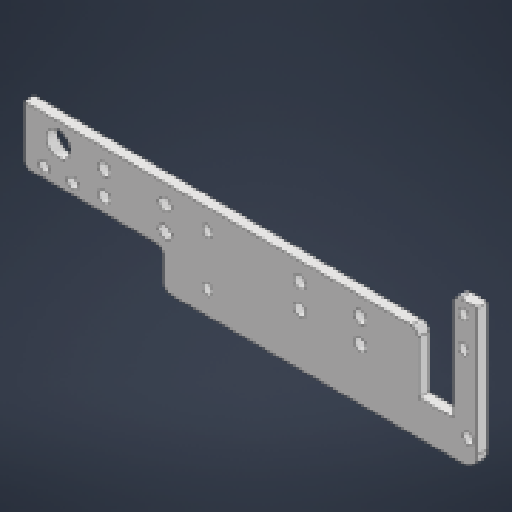
# Autodesk Inventor part: 外宽挤压
Saved by Autodesk Inventor 2025 (Build 290162000, 162)
## iProperties
Created: 2026-04-26
Part Number: 外宽挤压
Material: 常规
Document SubType Name: Modeling
Designer: XH
Density: 1 g/cm^3
Appearance: 默认
Author: XH
Autodesk Inventor part; units mm, degrees
ref_plane "YZ Plane" through (0, 0, 0) normal (1, 0, 0) x (0, 1, 0)
ref_plane "XZ Plane" through (0, 0, 0) normal (0, 1, 0) x (-1, 0, 0)
ref_plane "XY Plane" through (0, 0, 0) normal (0, 0, 1) x (1, 0, 0)
sketch "草图1" plane through (0, 0, 0) normal (0, 0, 1) x (1, 0, 0)
  line L0 (-43.79, -13.889) -> (86.21, -13.889)
  line L1 (86.21, -13.889) -> (86.21, 16.111)
  line L2 (86.21, 16.111) -> (-43.79, 16.111)
  line L3 (-43.79, 16.111) -> (-43.79, -13.889)
  dimension "d3" = 130
  dimension "d4" = 30
  constraints: 8 end point, 2 parallel, 1 horizontal, 1 perpendicular
  measures "d3" distance of L0.start L0.end
  measures "d4" distance of L0.end L1.end
extrude "拉伸1" add sketch "草图1" along normal blind 3
sketch "草图2" plane through (0, 0, 3) normal (0, 0, 1) x (1, 0, 0)
  line L0 (86.21, 16.111) -> (-43.79, 16.111) projected
  line L1 (69.2643, 16.111) -> (79.2643, 16.111)
  line L2 (79.2643, 16.111) -> (79.2643, -3.889)
  line L3 (79.2643, -3.889) -> (69.2643, -3.889)
  line L4 (69.2643, -3.889) -> (69.2643, 16.111)
  point P0 (0, 0)
  dimension "d5" = 10
  dimension "d6" = 20
  constraints: 8 end point, 2 parallel, 1 horizontal, 1 perpendicular, 1 point on line
  measures "d5" distance of L2.end L3.end
  measures "d6" distance of L1.end L2.end
extrude "拉伸2" cut sketch "草图2" against normal blind 3
fillet "圆角1" radius 2 2 edges at (69.2643, 16.111, 1.5) (79.2643, 16.111, 1.5)
sketch "草图3" plane through (0, 0, 3) normal (0, 0, 1) x (1, 0, 0)
  line L0 (-43.79, 16.111) -> (-43.79, -13.889) projected
  line L1 (-43.79, -13.889) -> (-3.79, -13.889)
  line L2 (-3.79, -13.889) -> (-3.79, 4.111)
  line L3 (-3.79, 4.111) -> (-43.79, 4.111)
  line L4 (-43.79, 4.111) -> (-43.79, -13.889)
  point P0 (0, 0)
  dimension "d10" = 40
  dimension "d11" = 18
  constraints: 8 end point, 2 parallel, 1 horizontal, 1 perpendicular
  measures "d10" distance between parallel lines of L2 L0
  measures "d11" distance between parallel lines of L1 L3
extrude "拉伸3" cut sketch "草图3" against normal blind 3
fillet "圆角2" radius 2 2 edges at (-3.79, 4.111, 1.5) (-3.79, -13.889, 1.5)
fillet "圆角3" radius 2 1 edges at (-43.79, 4.111, 1.5)
move faces "移动1" translate (0, 10.75, 0) faces at (84.5614, 16.111, 1)
fillet "圆角4" radius 4.25 1 edges at (86.21, -13.889, 1.5)
move faces "移动2" translate (0, -7.25, 0) faces at (-17.79, 4.111, 1)
sketch "草图4" plane through (0, 0, 0) normal (0, 0, -1) x (-1, 0, 0)
  line L0 (-0.892, -15.4705) -> (-0.8856, 17.0295) projected
  line L1 (-16.692, -15.4674) -> (-16.6856, 17.0326) projected
  line L2 (-0.889, 0) -> (-16.689, 0.0031)
  line L3 (-8.789, -13.6529) -> (-8.789, 16.111)
  line L4 (-67.2643, 16.111) -> (43.79, 16.111) projected
  circle A0 centre (-8.789, -7.1669) radius 1.55
  circle A1 centre (-8.7862, 7.17) radius 1.55
  point P0 (0, 0)
  point P1 (-8.789, 0.0016)
  dimension "d23" = 3.1
  constraints: 5 point on line, 4 end point, 2 centre point, 1 midpoint, 1 perpendicular, 1 symmetric about line, 1 vertical, 1 other
  measures "d23" diameter of A0
extrude "拉伸4" cut sketch "草图4" against normal blind 10 contours A1 L3 | L3 A1 | A0 L3 | L3 A0
sketch "草图5" plane through (0, 0, 0) normal (0, 0, -1) x (-1, 0, 0)
  circle A0 centre (-83.46, -6.8603) radius 1.5 projected
  circle A1 centre (-82.1717, 14.6045) radius 1.5 projected
  circle A2 centre (-82.1717, 23.2524) radius 1.5 projected
  line L0 (-67.41, 27.075) -> (-67.41, 17.075) projected
  line L1 (-86.21, 27.075) -> (-67.41, 27.075) projected
  line L2 (-86.21, -11.1435) -> (-86.21, 27.075) projected
  line L3 (-80.71, -11.1435) -> (-86.21, -11.1435) projected
  line L4 (-80.71, 10.8565) -> (-80.71, -11.1435) projected
  line L5 (-77.71, 10.8565) -> (-80.71, 10.8565) projected
  line L6 (-77.71, 25.075) -> (-77.71, 10.8565) projected
  line L7 (-72.41, 25.075) -> (-77.71, 25.075) projected
  line L8 (-72.41, 17.075) -> (-72.41, 25.075) projected
  line L9 (-67.41, 17.075) -> (-72.41, 17.075) projected
  point P0 (0, 0)
extrude "拉伸5" cut sketch "草图5" against normal blind 10 contours A0 | A1 | A2
sketch "草图6" plane through (0, 0, 3) normal (0, 0, 1) x (1, 0, 0)
  line L0 (-43.79, 16.111) -> (-43.79, -1.139) projected
  line L1 (-43.79, 7.486) -> (-28.8544, 7.486)
  circle A0 centre (-33.8796, 7.486) radius 3.5
  point P0 (0, 0)
  dimension "d28" = 7
  constraints: 2 end point, 1 centre point, 1 horizontal, 1 midpoint, 1 point on line
  measures "d28" diameter of A0
extrude "拉伸6" cut sketch "草图6" against normal blind 10
move faces "移动3" translate (0, -3, 0) faces at (30.2462, 16.111, 1)
sketch "草图7" plane through (0, 0, 3) normal (0, 0, 1) x (1, 0, 0)
  line L0 (-24.0244, 11.792) -> (-17.652, 11.7933) projected
  line L1 (-24.0214, -3.208) -> (-24.0244, 11.792) projected
  line L2 (-17.649, -3.2067) -> (-24.0214, -3.208) projected
  line L3 (-17.652, 11.7933) -> (-17.649, -3.2067) projected
  line L4 (-0.0244, 11.7968) -> (-6.3968, 11.7955) projected
  line L5 (-6.3939, -3.2045) -> (-6.3968, 11.7955) projected
  line L6 (-6.3939, -3.2045) -> (-0.0214, -3.2032) projected
  line L7 (-0.0214, -3.2032) -> (-0.0244, 11.7968) projected
  line L8 (31.9024, 11.6365) -> (38.2749, 11.6378) projected
  line L9 (31.9054, -3.3635) -> (31.9024, 11.6365) projected
  line L10 (38.2779, -3.3622) -> (31.9054, -3.3635) projected
  line L11 (38.2749, 11.6378) -> (38.2779, -3.3622) projected
  line L12 (55.9054, -3.3587) -> (55.9024, 11.6413) projected
  line L13 (55.9024, 11.6413) -> (49.53, 11.64) projected
  line L14 (49.533, -3.36) -> (49.53, 11.64) projected
  line L15 (49.533, -3.36) -> (55.9054, -3.3587) projected
  line L16 (55.9054, -3.3587) -> (55.9024, 11.6413) projected
  line L17 (-20.8382, 11.7926) -> (-20.8352, -3.2074)
  line L18 (-3.2106, 11.7961) -> (-3.2077, -3.2039)
  line L19 (35.0887, 11.6371) -> (35.0916, -3.3629)
  line L20 (52.7162, 11.6406) -> (52.7192, -3.3594)
  circle A0 centre (-20.8374, 7.7585) radius 1.75
  line L21 (-24.0229, 4.292) -> (-17.6505, 4.2933)
  circle A1 centre (-20.836, 0.8268) radius 1.75
  circle A2 centre (-3.2098, 7.7585) radius 1.75
  circle A3 centre (-3.2085, 0.8268) radius 1.75
  circle A4 centre (52.7184, 0.8268) radius 1.75
  circle A5 centre (52.717, 7.7585) radius 1.75
  circle A6 centre (35.0908, 0.8268) radius 1.75
  circle A7 centre (35.0894, 7.7585) radius 1.75
  ellipse E0 centre (-20.7244, 7.7585) end of major axis (-18.9875, 7.9728) minor radius 1.7495 projected
  ellipse E1 centre (-20.723, 0.9823) end of major axis (-18.9862, 1.1966) minor radius 1.7495 projected
  ellipse E2 centre (-3.3416, 7.7585) end of major axis (-1.6048, 7.9728) minor radius 1.7495 projected
  ellipse E3 centre (-3.3408, 0.9823) end of major axis (-1.604, 1.1966) minor radius 1.7495 projected
  ellipse E4 centre (52.5852, 7.603) end of major axis (54.322, 7.8173) minor radius 1.7495 projected
  ellipse E5 centre (52.586, 0.8268) end of major axis (54.3229, 1.0411) minor radius 1.7495 projected
  ellipse E6 centre (35.2025, 7.603) end of major axis (36.9393, 7.8173) minor radius 1.7495 projected
  ellipse E7 centre (35.2038, 0.8268) end of major axis (36.9406, 1.0411) minor radius 1.7495 projected
  point P0 (0, 0)
  dimension "d34" = 3.5
  dimension "d35" = 3.5
  dimension "d37" = 3.5
  dimension "d38" = 3.5
  constraints: 10 end point, 10 midpoint, 8 centre point, 7 point on line, 6 horizontal alignment, 1 symmetric about line, 1 other
  measures "d34" diameter of A0
  measures "d35" diameter of A2
  measures "d37" diameter of A5
  measures "d38" diameter of A7
extrude "拉伸7" cut sketch "草图7" against normal blind 10 contours A0 E0 L17 | L17 E0 A0 | E0 A0 L17 | L17 E0 | L17 E0 A0 | A1 E1 L17 | L17 E1 A1 | A1 E1 L17 | L17 E1 A1 | A2 L18 E2 | L18 E2 A2 | E2 L18 | L18 E2 A2 | A3 E3 L18 | L18 E3 A3 | L18 A2 E2 | E3 A3 L18 | L18 A3 E3 | A7 E6 L19 | L19 E6 A7 | E6 A7 L19 | L19 A7 E6 | A6 L19 E7 | L19 E7 A6 | E7 L19 | L19 E7 A6 | A6 E7 L19 | A4 E5 L20 | L20 E5 A4 | A5 E4 L20 | L20 E4 A5 | E5 A4 L20 | L20 E5 | E4 A5 L20 | L20 A5 E4 | E5 A4 L20 picked at (-21.8423, -0.4354) picked at (-20.7011, -0.8099) picked at (-20.7063, 1.4487) picked at (-21.2532, 0.4647) picked at (-3.3265, -0.8128) picked at (-2.2025, -0.4239) picked at (-3.3508, 1.4462) picked at (-3.0699, 0.3785) picked at (35.3084, 9.4373) picked at (34.1133, 9.0435) picked at (35.2194, 7.1366) picked at (34.959, 8.2119) picked at (53.6916, 9.0354) picked at (52.5826, 9.4392) picked at (52.8477, 8.2095) picked at (52.575, 7.1391)
sketch "草图8" plane through (0, 0, 3) normal (0, 0, 1) x (1, 0, 0)
  circle A0 centre (-37.9757, -0.1375) radius 1.5 projected
  circle A1 centre (-29.7757, -0.1333) radius 1.5 projected
  point P0 (0, 0)
extrude "拉伸8" cut sketch "草图8" against normal blind 10
